skadis_nut_left (Autodesk Fusion 360 design; units mm, degrees)
part number: 2026-09-06-14-40-21-794
Autodesk Fusion 360 part; units mm, degrees
sketch "Plate" plane through (0, 0, 0) normal (0, 1, 0) x (1, 0, 0)
  line L0 (0, 0) -> (11, 0)
  line L1 (11, 0) -> (11, -48)
  line L2 (11, -48) -> (0, -48)
  line L3 (0, -48) -> (0, 0)
  dimension "d76" = 11
  dimension "d77" = 48
  constraint coincident L0.start L3.end
  constraint horizontal L0
  constraint horizontal L2
  constraint vertical L1
  constraint vertical L3
  measures "d76" horizontal distance of L0.start L1.end
  measures "d77" vertical distance of L0.start L1.end
extrude "Plate (1)" add sketch "Plate" along normal mid plane 33 from surface at 4.5
sketch "Hook profile" plane through (0, 0, 0) normal (0, 1, 0) x (1, 0, 0)
  line L0 (0, -46) -> (-8.3, -46)
  line L1 (-8.3, -46) -> (-8.3, -29)
  line L2 (-8.3, -29) -> (-5.3, -29)
  line L3 (-5.3, -29) -> (-3.8, -30.5)
  line L4 (-3.8, -30.5) -> (-3.8, -41)
  line L5 (-3.8, -41) -> (0, -41)
  line L6 (0, -41) -> (0, -46)
  dimension "d81" = 46
  dimension "d82" = 8.3
  dimension "d83" = 3.8
  dimension "d84" = 5
  dimension "d85" = 10.5
  dimension "d86" = 1.5
  dimension "d87" = 1.5
  constraint horizontal L0
  constraint horizontal L2
  constraint horizontal L5
  constraint vertical L1
  constraint vertical L4
  constraint vertical L6
  constraint coincident origin L6
  measures "d81" vertical distance of origin L0.start
  measures "d82" horizontal distance of L0.start L0.end
  measures "d83" horizontal distance of L4.end L5.end
  measures "d84" vertical distance of L0.start L5.end
  measures "d85" vertical distance of L3.end L4.end
  measures "d86" horizontal distance of L2.end L3.end
  measures "d87" vertical distance of L2.end L3.end
extrude "Hook profile (1)" add sketch "Hook profile" along normal mid plane 2.4
pattern_linear "Hook rows" count 2 spacing 25.4 along (0, 0, -1) count 3 spacing 0 along (0, 0, 1) of "Hook profile (1)"
sketch "Nut channel" plane through (0, 0, 0) normal (0, 1, 0) x (1, 0, 0)
  line L0 (9, -20.3) -> (12, -20.3)
  line L1 (12, -20.3) -> (12, -27.7)
  line L2 (12, -27.7) -> (9, -27.7)
  line L3 (9, -27.7) -> (9, -20.3)
  dimension "d94" = 12
  dimension "d95" = 20.3
  dimension "d96" = 3
  dimension "d97" = 7.4
  constraint horizontal L0
  constraint horizontal L2
  constraint vertical L1
  constraint vertical L3
  measures "d94" horizontal distance of origin L0.end
  measures "d95" vertical distance of origin L0.end
  measures "d96" horizontal distance of L0.start L0.end
  measures "d97" vertical distance of L0.end L1.end
extrude "Nut channel (1)" cut sketch "Nut channel" along normal mid plane 19.4 from surface at 7.52
sketch "Screw relief" plane through (0, 0, 0) normal (0, 1, 0) x (1, 0, 0)
  line L0 (-1, -21.6) -> (12, -21.6)
  line L1 (12, -21.6) -> (12, -26.4)
  line L2 (12, -26.4) -> (-1, -26.4)
  line L3 (-1, -26.4) -> (-1, -21.6)
  dimension "d101" = 12
  dimension "d102" = 21.6
  dimension "d103" = 13
  dimension "d104" = 4.8
  constraint horizontal L0
  constraint horizontal L2
  constraint vertical L1
  constraint vertical L3
  measures "d101" horizontal distance of origin L0.end
  measures "d102" vertical distance of origin L0.end
  measures "d103" horizontal distance of L0.start L0.end
  measures "d104" vertical distance of L0.end L1.end
extrude "Screw relief (1)" cut sketch "Screw relief" along normal mid plane 16.8 from surface at 7.52
equation "bracketWidth = 24.0 mm" comment "bracket width across the upright"
equation "plateHeight = 48.0 mm" comment "plate height"
equation "plateInboardExtension = 9.0 mm" comment "extra plate toward the desk centre, where the channel reaches"
equation "boardThickness = 6.0 mm" comment "measured SKADIS panel thickness"
equation "screwLength = 15.0 mm" comment "measured decorative M4 screw"
equation "screwDiameter = 4.0 mm" comment "M4 shank"
equation "screwClearance = 0.8 mm" comment "slack around the shank"
equation "screwTipClearance = 2.2 mm" comment "tip stops this short of the plate's back face"
equation "screwSlotWidth = screwDiameter + screwClearance" comment "screw relief slot height"
equation "nutAcrossFlats = 7.0 mm" comment "M4 square nut across flats"
equation "nutThickness = 2.2 mm" comment "M4 square nut thickness"
equation "nutChannelClearance = 0.4 mm" comment "slack around the nut in its channel"
equation "nutProud = 0.2 mm" comment "nut stands out of the pocket to be clamped"
equation "nutPocketDepth = nutThickness - nutProud" comment "channel depth"
equation "nutChannelHeight = nutAcrossFlats + nutChannelClearance" comment "channel height; under the nut's diagonal so it cannot turn"
equation "plateThickness = screwLength - boardThickness - nutProud + screwTipClearance" comment "derived: deep enough to swallow the screw"
equation "mountTravel = 12.0 mm" comment "left-right adjustment"
equation "nutChannelLength = mountTravel + nutAcrossFlats + nutChannelClearance" comment "channel length along the plate"
equation "screwSlotLength = mountTravel + screwSlotWidth" comment "relief slot length along the plate"
equation "topMountZ = 24.0 mm" comment "top channel centre"
equation "mountOffsetY = 7.52 mm" comment "channel centre on the board's grid"
equation "slotOvershoot = 1.0 mm" comment "cuts reach past the faces they cut"
equation "slotWidth = 3.2 mm" comment "measured upright slot width"
equation "slotPitchVertical = 25.4 mm" comment "1 inch, measured"
equation "faceMetalThickness = 2.0 mm" comment "upright face metal"
equation "hookTabWidth = slotWidth - 0.8 mm" comment "blade width through the slot"
equation "hookThroat = faceMetalThickness + 1.8 mm" comment "gap behind the plate"
equation "hookNeckHeight = 5.0 mm" comment "bears on the slot bottom edge"
equation "hookLipThickness = 4.5 mm" comment "lip behind the upright face"
equation "hookLipDrop = 12.0 mm" comment "engagement below the neck"
equation "hookLipChamfer = 1.5 mm" comment "lead-in past slot burrs"
equation "topHookNeckTop = plateHeight - 2 mm" comment "top hook row"
equation "hookRows = 2" comment "hook rows (pattern count)"
equation "d76 = plateThickness"
equation "d77 = plateHeight"
equation "d78 = plateInboardExtension / 2"
equation "d79 = bracketWidth + plateInboardExtension"
equation "d81 = topHookNeckTop"
equation "d82 = hookThroat + hookLipThickness"
equation "d83 = hookThroat"
equation "d84 = hookNeckHeight"
equation "d85 = hookLipDrop - hookLipChamfer"
equation "d86 = hookLipChamfer"
equation "d87 = hookLipChamfer"
equation "d88 = hookTabWidth"
equation "d90 = hookRows"
equation "d92 = -slotPitchVertical"
equation "d94 = plateThickness + slotOvershoot"
equation "d95 = topMountZ - nutChannelHeight / 2"
equation "d96 = nutPocketDepth + slotOvershoot"
equation "d97 = nutChannelHeight"
equation "d98 = mountOffsetY"
equation "d99 = nutChannelLength"
equation "d101 = plateThickness + slotOvershoot"
equation "d102 = topMountZ - screwSlotWidth / 2"
equation "d103 = plateThickness + 2 * slotOvershoot"
equation "d104 = screwSlotWidth"
equation "d105 = mountOffsetY"
equation "d106 = screwSlotLength"
named bodies: "skadis_nut_left"
